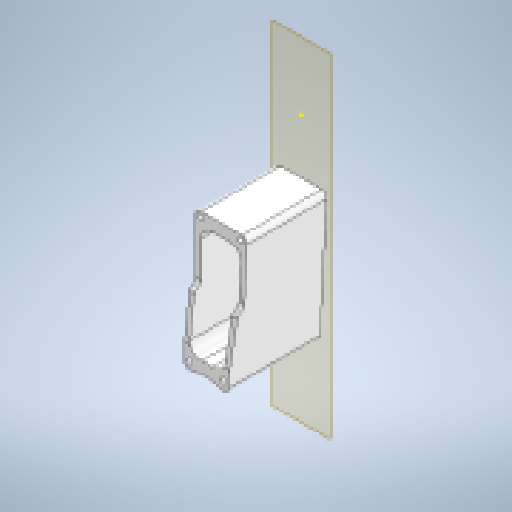
# Autodesk Inventor part: suzikai_3204
Saved by Autodesk Inventor 2024 (Build 280153000, 153)
## iProperties
Created: 2024-01-03
Part Number: suzikai_3204
Material: ABS プラスチック
Document SubType Name: Modeling
Designer: right
Density: 1.06 g/cm^3
Appearance: 滑らか - 白
Mass: 14.1558 g
Surface Area: 92.6475 cm^2
Volume: 13.3545 cm^3
Author: right
Autodesk Inventor part; units mm, degrees
ref_plane "YZ Plane" through (0, 0, 0) normal (1, 0, 0) x (0, 1, 0)
ref_plane "作業平面3" through (-10.19298, -96.69298, 34.9) normal (0, 0, 1) x (0.9997018, 0.0244208, 0)
sketch "スケッチ1" plane through (0, 0, 0) normal (0, 0, 1) x (1, 0, 0)
  arc A0 (6.898427, -72.853339) -> (-10, -72.375485) centre (-2, -88.5) ccw
  circle A1 centre (-8, -68.5) radius 1.1
  circle A2 centre (5, -68.5) radius 1.1
  circle A3 centre (5.5, -57.125) radius 1.1
  circle A4 centre (-8, -57.125) radius 1.1
  circle A5 centre (-8, -45.75) radius 1.1
  circle A6 centre (6, -45.75) radius 1.1
  circle A7 centre (6.5, -34.375) radius 1.1
  circle A8 centre (-8, -34.375) radius 1.1
  circle A9 centre (-8, -23) radius 1.1
  circle A10 centre (7, -23) radius 1.1
  line L0 (-11.062221, -21) -> (8.846468, -21)
  line L1 (-10, 18) -> (-10, -88.5)
  line L2 (5.987216, -88.952087) -> (9.996804, -18.113022)
  line L3 (8.432513, -45.75) -> (-10, -45.75)
  circle A11 centre (-8, -68.5) radius 1
  circle A12 centre (5, -68.5) radius 1
  circle A13 centre (5.5, -57.125) radius 1
  circle A14 centre (-8, -57.125) radius 1
  point P0 (0, 0)
  point P1 (-9.1, -45.75)
  point P2 (4.9, -45.75)
  point P3 (7.1, -45.75)
  point P4 (-6.9, -45.75)
  dimension "d0" = 2
  dimension "d10" = 2
  dimension "d11" = 2
  dimension "d12" = 2
  dimension "d13" = 2
  constraints: 4 centre point, 4 coincident, 4 end point, 3 point on line, 1 horizontal, 1 perpendicular
  measures "d0" distance from line of A9.centre L0
  measures "d10" diameter of A11
  measures "d11" diameter of A12
  measures "d12" diameter of A13
  measures "d13" diameter of A14
extrude "押し出し1" add sketch "スケッチ1" along normal up to surface (34.9 mm away) contours A0 L1 L3 A5 A6 L2 | A6 L3 | L3 A5 | A1 | A2 | A3 | A4 | A13 | A14 picked at (6.044197, -46.113993) picked at (-7.955803, -46.113993)
ref_plane "作業平面1" through (102.660398, 0, 0) normal (0, 0, 1) x (1, 0, 0)
sketch "スケッチ2" plane through (0, 0, 0) normal (0, 0, 1) x (1, 0, 0)
  line L0 (8.432513, -45.75) -> (-10, -45.75)
  circle A0 centre (-8, -34.375) radius 1.1
  circle A1 centre (7, -23) radius 1.1
  circle A2 centre (5, -68.5) radius 1.1
  circle A3 centre (5.5, -57.125) radius 1.1
  circle A4 centre (6.5, -34.375) radius 1.1
  circle A5 centre (-8, -23) radius 1.1
  circle A6 centre (-8, -68.5) radius 1.1
  circle A7 centre (-8, -57.125) radius 1.1
  arc A8 (-6.25, 0.323982) -> (-6, 1.292228) centre (-8, 1.292228) ccw
  line L1 (-6, 1.292228) -> (-6, 6.208497)
  arc A9 (-6, 16.791503) -> (-6, 6.208497) centre (0, 11.5) ccw
  line L2 (-6, 16.791503) -> (-6, 18)
  arc A10 (-6, 18) -> (-10, 18) centre (-8, 18) ccw
  line L3 (-10, 18) -> (-10, -88.5)
  arc A11 (-10, -88.5) -> (5.987216, -88.952087) centre (-2, -88.5) ccw
  line L4 (5.987216, -88.952087) -> (9.996804, -18.113022)
  arc A12 (9.996804, -18.113022) -> (8, -16) centre (8, -18) ccw
  line L5 (8, -16) -> (-4, -16)
  arc A13 (-6, -14) -> (-4, -16) centre (-4, -14) ccw
  line L6 (-6, -14) -> (-6, -7.213616)
  arc A14 (-6, -7.213616) -> (-6.25, -6.24537) centre (-8, -7.213616) ccw
  arc A15 (-6.5, -5.277124) -> (-6.25, -6.24537) centre (-4.5, -5.277124) ccw
  line L7 (-6.5, -5.277124) -> (-6.5, -0.644264)
  arc A16 (-6.25, 0.323982) -> (-6.5, -0.644264) centre (-4.5, -0.644264) ccw
  circle A17 centre (-8, -18) radius 1.1
  circle A18 centre (-8, 18) radius 1.1
  circle A19 centre (8, -18) radius 1.1
  circle A20 centre (-6.242641, -84.257359) radius 1.1
  circle A21 centre (-2, -82.5) radius 1.1
  circle A22 centre (2.242641, -84.257359) radius 1.1
  circle A23 centre (4, -88.5) radius 1.1
  circle A24 centre (2.242641, -92.742641) radius 1.1
  circle A25 centre (-2, -94.5) radius 1.1
  circle A26 centre (-6.242641, -92.742641) radius 1.1
  circle A27 centre (-8, -88.5) radius 1.1
  circle A28 centre (-2, -88.5) radius 4
  line L8 (9.5, -20) -> (-9.5, -20)
  line L9 (-10, -21) -> (9.833397, -21)
  arc A29 (4.951888, -27.613022) -> (2.955084, -25.5) centre (2.955084, -27.5) ccw
  line L10 (4.951888, -27.613022) -> (2.876327, -64.282828)
  arc A30 (0.64446, -66.155944) -> (2.876327, -64.282828) centre (0.879523, -64.169806) ccw
  arc A31 (0.64446, -66.155944) -> (-3.377551, -66.04221) centre (-2, -88.5) ccw
  arc A32 (-5.5, -64.045961) -> (-3.377551, -66.04221) centre (-3.5, -64.045961) ccw
  line L11 (-5.5, -64.045961) -> (-5.5, -27.5)
  arc A33 (-3.5, -25.5) -> (-5.5, -27.5) centre (-3.5, -27.5) ccw
  line L12 (-3.5, -25.5) -> (2.955084, -25.5)
  circle A34 centre (6.5, -34.375) radius 1
  circle A35 centre (7, -23) radius 1
  circle A36 centre (-8, -34.375) radius 1
  circle A37 centre (-8, -23) radius 1
  point P0 (0, 0)
  dimension "d3" = 2
  dimension "d14" = 2
  dimension "d15" = 2
  dimension "d16" = 2
  dimension "d17" = 2
  constraints: 4 centre point, 4 coincident, 2 end point, 2 point on line, 1 parallel
  measures "d3" distance from line of A5.centre L9
  measures "d14" diameter of A34
  measures "d15" diameter of A35
  measures "d16" diameter of A36
  measures "d17" diameter of A37
ref_plane "作業平面2" through (-11.190434, -20.698035, 30.5) normal (0, 0, 1) x (1, 0, 0)
extrude "押し出し2" add sketch "スケッチ2" along normal up to surface (30.5 mm away) contours L0 L10 A29 L12 A33 L11 L3 L9 L4 | L0 L11 A33 L12 A29 L10 | A0 | A1 | A4 | A5 | A34 | A36
sketch "スケッチ3" plane through (0, 0, 0) normal (0, 0, -1) x (-1, 0, 0)
  point P0 (0, 0)
sketch "スケッチ4" plane through (0, 0, 0) normal (0, 0, -1) x (-1, 0, 0)
  line L0 (10, -21) -> (10, -72.375485)
  line L1 (10, -45.75) -> (10, -21)
  arc A0 (10, -72.375485) -> (-6.898427, -72.853339) centre (2, -88.5) ccw
  line L2 (-6.898427, -72.853339) -> (-9.833397, -21)
  line L3 (-9.833397, -21) -> (-8.432513, -45.75)
  line L4 (-9.833397, -21) -> (10, -21)
  arc A1 (5.5, -66.273889) -> (-9.123034, -68.941674) centre (2, -88.5) ccw
  line L5 (5.5, -66.273889) -> (5.5, -25.5)
  line L6 (5.5, -25.5) -> (-5.071488, -25.5)
  line L7 (-5.071488, -25.5) -> (-2.405618, -72.59904)
  line L8 (-8.432513, -45.75) -> (-6.898427, -72.853339)
  line L9 (10, -72.375485) -> (10, -45.75)
  point P0 (0, 0)
  point P1 (-2.750425, -66.507195)
  dimension "d6" = 4.5
  constraints: 6 end point, 2 point on circle, 1 centre point, 3 other
  measures "d6" distance between parallel lines of L0 L5
extrude "押し出し3" cut sketch "スケッチ4" against normal through all contours L7 L6 L5 A1
fillet "フィレット1" radius 2 12 edges at (-5.5, -25.5, 15.25) (5.0715, -25.5, 15.25) (2.7504, -66.5072, 17.45) (-5.5, -66.2739, 17.45) (-10, -21, 15.25) (9.8334, -21, 15.25) (6.8984, -72.8533, 17.45) (-10, -72.3755, 17.45) (-7.75, -45.75, 30.5) (6.1789, -45.75, 30.5) (6.1789, -45.75, 34.9) (-7.75, -45.75, 34.9)
sketch "スケッチ5" plane through (7.065375, -69.903792, 34.9) normal (0.998402, -0.0565109, 0) x (0, 0, -1)
  line L0 (0, 5.893801) -> (-1.5, 5.893801)
  line L1 (4.4, 43.481475) -> (2.9, 43.481475)
  line L2 (0, 5.893801) -> (4.4, 43.481475)
  ellipse E0 centre (2, 22.18925) end of major axis (2, 24.192452) minor radius 2 (2, 24.192452) -> (0, 22.18925) ccw
  line L3 (0, 22.18925) -> (0, 0)
  line L4 (34.9, 0) -> (0, 0)
  line L5 (34.9, 0) -> (34.9, 46.865662)
  line L6 (4.4, 46.865662) -> (34.9, 46.865662)
  line L7 (4.4, 46.865662) -> (4.4, 26.195653)
  ellipse E1 centre (2.4, 26.195653) end of major axis (2.4, 24.192452) minor radius 2 (2.4, 24.192452) -> (4.4, 26.195653) ccw
  line L8 (2.4, 24.192452) -> (2, 24.192452)
  point P0 (34.9, 69.392813)
  point P1 (2.142034, 24.192452)
  point P2 (0, 5.893801)
  constraints: 2 end point, 2 other
extrude "押し出し4" cut sketch "スケッチ5" against normal through all contours L3 E0 L8 L2 | L2 L7 E1 L8
fillet "フィレット2" radius 2 2 edges at (6.1789, -45.75, 32.7729) (-7.75, -45.75, 32.865)
sketch "スケッチ6" plane through (0, 0, 0) normal (0, 0, -1) x (-1, 0, 0)
  line L0 (-4.272707, -66.155944) -> (-6.573889, -25.5)
  line L1 (-7.065375, -69.903792) -> (-9.713797, -23.113022)
  arc A0 (-2.876327, -64.282828) -> (-0.64446, -66.155944) centre (-0.879523, -64.169806) ccw
  arc A1 (-4.453656, -62.959039) -> (-0.64446, -66.155944) centre (-1.04565, -62.766141) ccw
  arc A2 (-2.955084, -25.5) -> (-4.951888, -27.613022) centre (-2.955084, -27.5) ccw
  arc A3 (-2.955084, -25.5) -> (-6.369387, -29.113022) centre (-2.955084, -28.919768) ccw
  line L2 (-2.955084, -25.5) -> (3.5, -25.5) construction
  arc A4 (7.4, -71.329094) -> (-4.361714, -71.661693) centre (2, -88.5) ccw construction
  line L3 (0.272458, -25.5) -> (2, -88.5) construction
  line L4 (-2.053122, -78.826728) -> (-4.951888, -27.613022)
  arc A5 (-2.955084, -25.5) -> (-4.951888, -27.613022) centre (-2.955084, -27.5) ccw
  line L5 (-2.955084, -25.5) -> (3.5, -25.5)
  arc A6 (5.5, -27.5) -> (3.5, -25.5) centre (3.5, -27.5) ccw
  line L6 (5.5, -27.5) -> (5.5, -78.61314)
  arc A7 (3.2, -80.590512) -> (5.5, -78.61314) centre (3.5, -78.61314) ccw
  arc A8 (3.2, -80.590512) -> (0.354945, -80.670965) centre (2, -88.5) ccw
  arc A9 (-2.053122, -78.826728) -> (0.354945, -80.670965) centre (-0.056319, -78.713706) ccw
  circle A10 centre (-7, -23) radius 1.1
  circle A11 centre (-5, -68.5) radius 1.1
  circle A12 centre (8, -23) radius 1.1
  circle A13 centre (8, -68.5) radius 1.1
  arc A14 (6, 1.292228) -> (6.25, 0.323982) centre (8, 1.292228) ccw
  arc A15 (6.5, -0.644264) -> (6.25, 0.323982) centre (4.5, -0.644264) ccw
  line L7 (6.5, -5.277124) -> (6.5, -0.644264)
  arc A16 (6.25, -6.24537) -> (6.5, -5.277124) centre (4.5, -5.277124) ccw
  arc A17 (6.25, -6.24537) -> (6, -7.213616) centre (8, -7.213616) ccw
  line L8 (6, -14) -> (6, -7.213616)
  arc A18 (4, -16) -> (6, -14) centre (4, -14) ccw
  line L9 (-8, -16) -> (4, -16)
  arc A19 (-8, -16) -> (-9.996804, -18.113022) centre (-8, -18) ccw
  line L10 (-5.987216, -88.952087) -> (-9.996804, -18.113022)
  arc A20 (-5.987216, -88.952087) -> (10, -88.5) centre (2, -88.5) ccw
  line L11 (10, 18) -> (10, -88.5)
  arc A21 (10, 18) -> (6, 18) centre (8, 18) ccw
  line L12 (6, 16.791503) -> (6, 18)
  arc A22 (6, 6.208497) -> (6, 16.791503) centre (0, 11.5) ccw
  line L13 (6, 1.292228) -> (6, 6.208497)
  circle A23 centre (8, -18) radius 1.1
  circle A24 centre (8, 18) radius 1.1
  circle A25 centre (-8, -18) radius 1.1
  circle A26 centre (6.242641, -84.257359) radius 1.1
  circle A27 centre (2, -82.5) radius 1.1
  circle A28 centre (-2.242641, -84.257359) radius 1.1
  circle A29 centre (-4, -88.5) radius 1.1
  circle A30 centre (-2.242641, -92.742641) radius 1.1
  circle A31 centre (2, -94.5) radius 1.1
  circle A32 centre (6.242641, -92.742641) radius 1.1
  circle A33 centre (8, -88.5) radius 1.1
  circle A34 centre (2, -88.5) radius 4
  line L14 (7, -26.085786) -> (7, -62.635152)
  line L15 (10, -23) -> (10, -69.421216)
  arc A35 (3.377551, -66.04221) -> (5.5, -64.045961) centre (3.5, -64.045961) ccw
  arc A36 (3.377551, -66.04221) -> (7, -62.635152) centre (3.586538, -62.635152) ccw
  arc A37 (5.5, -27.5) -> (3.5, -25.5) centre (3.5, -27.5) ccw
  arc A38 (7, -29) -> (3.5, -25.5) centre (3.5, -29) ccw
  point P0 (0, 0)
  point P1 (-8.389586, -46.508407)
  point P2 (3.416001, -66.044601)
  point P3 (-2.796312, -65.696482)
  point P4 (5.5, -65.461878)
  dimension "d21" = 3
  dimension "d24" = 3
  constraints: 8 point on circle, 8 tangent, 6 end point, 4 centre point, 3 point on line, 2 horizontal alignment, 2 midpoint, 1 parallel, 1 symmetric about line, 1 vertical
  measures "d21" distance from line of point (-8.39, -46.508) L0
  measures "d24" distance between parallel lines of L15 L14
extrude "押し出し5" cut sketch "スケッチ6" against normal through all contours L0 A3 A2 L4 A1 | L4 A0 A1 | A38 L14 A36 L6 A6 | L6 A36 A35
equation "\"d21\" = d24"
